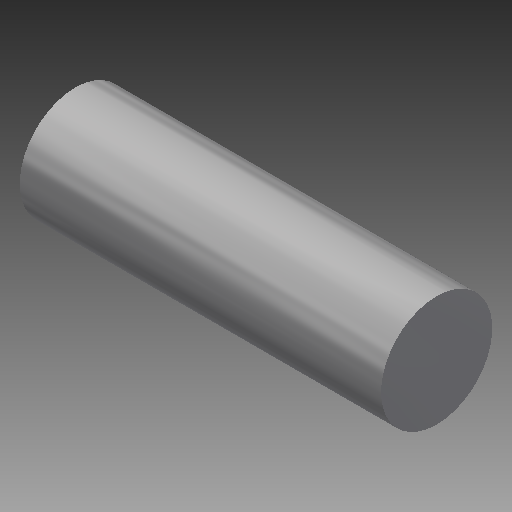
# Autodesk Inventor part: Shaft
Saved by Autodesk Inventor 2017 SP1 (Build 210196100, 196)
## iProperties
Created: 2017-06-15
Part Number: Shaft
Material: Steel
Document SubType Name: Modeling
Designer: RMcComber
Density: 1 g/cm^3
Appearance: Steel
CustomPartVersion: 1
Author: RMcComber
Autodesk Inventor part; units mm, degrees
ref_plane "Start Plane" through (0, 0, 0) normal (1, 0, 0) x (0, 1, 0)
ref_plane "XZ Plane" through (0, 0, 0) normal (0, 1, 0) x (-1, 0, 0)
ref_plane "XY Plane" through (0, 0, 0) normal (0, 0, 1) x (1, 0, 0)
sketch "Main Sketch" plane through (0, 0, 0) normal (0, 0, 1) x (1, 0, 0)
  line L0 (0, 0) -> (26, 0)
  line L1 (0, 0) -> (0, 4)
  line L2 (26, 4) -> (26, 0)
  line L3 (0, 4) -> (26, 4)
  dimension "d3" = 8
  constraints: 8 end point, 3 horizontal, 2 vertical
  measures "d3" diameter of L3 L0
revolve "Revolution1" add sketch "Main Sketch" angle 360 about axis through (0, 0, 0) along (1, 0, 0)
body "Solid1"
